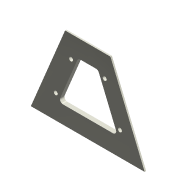
# Autodesk Inventor part: Stage2
Saved by Autodesk Inventor 2018.2 (Build 222227000, 227)
## iProperties
Created: 2018-11-01
Part Number: Stage2
Material: ABS-Kunststoff
Document SubType Name: Modeling
Designer: M.Knabel
Density: 1.06 g/cm^3
Appearance: Glatt - Elfenbein
Mass: 26.953 g
Surface Area: 131.178 cm^2
Volume: 25.4274 cm^3
Author: M.Knabel
Autodesk Inventor part; units mm, degrees
ref_plane "YZ Plane" through (0, 0, 0) normal (1, 0, 0) x (0, 1, 0)
ref_plane "XZ Plane" through (0, 0, 0) normal (0, 1, 0) x (-1, 0, 0)
ref_plane "XY Plane" through (0, 0, 0) normal (0, 0, 1) x (1, 0, 0)
sketch "Skizze1" plane through (0, 0, 0) normal (0, 1, 0) x (-1, 0, 0)
  line L0 (-22.75, 41.5) -> (22.75, 41.5)
  line L1 (22.75, 41.5) -> (57.1297, -41.5)
  line L2 (57.1297, -41.5) -> (-57.1297, -41.5)
  line L3 (-57.1297, -41.5) -> (-22.75, 41.5)
  line L4 (79.9816, 0) -> (-79.9816, 0) construction
  line L5 (0, -58.1) -> (0, 58.1) construction
  point P0 (0, 0)
  dimension "d0" = 83
  dimension "d1" = 112.5
  dimension "d2" = 45.5
  constraints: 8 end point, 1 horizontal, 1 parallel, 2 other
  measures "d0" distance between parallel lines of L2 L0
  measures "d1" angle of L0 L3
  measures "d2" distance of L0.start L0.end
extrude "Extrusion1" add sketch "Skizze1" along normal blind 6
sketch "Skizze2" plane through (0, 6, 0) normal (0, 1, 0) x (1, 0, 0)
  line L0 (-22.75, -41.5) -> (22.75, -41.5) projected
  line L1 (22.75, -41.5) -> (57.1297, 41.5) projected
  line L2 (57.1297, 41.5) -> (-57.1297, 41.5) projected
  line L3 (-57.1297, 41.5) -> (-22.75, -41.5) projected
  line L4 (-49.6467, 36.5) -> (49.6467, 36.5)
  line L5 (49.6467, 36.5) -> (19.4091, -36.5)
  line L6 (19.4091, -36.5) -> (-19.4091, -36.5)
  line L7 (-19.4091, -36.5) -> (-49.6467, 36.5)
  point P0 (0, 0)
  dimension "d5" = 5
  constraints: 8 end point, 3 other
  measures "d5" distance between parallel lines of L2 L4
extrude "Extrusion2" cut sketch "Skizze2" against normal blind 3.5
sketch "Skizze4" plane through (0, 6, 0) normal (0, 1, 0) x (1, 0, 0)
  line L0 (58.5766, 41.5) -> (-55.8797, 41.5) construction
  line L1 (-55.8797, 41.5) -> (-21.5, -41.5) construction
  line L2 (-21.5, -41.5) -> (24.1969, -41.5) construction
  line L3 (57.1297, 41.5) -> (22.75, -41.5) construction
  line L4 (22.4292, -40.7678) -> (56.8089, 42.2322) construction
  line L5 (-29.4207, 23.8207) -> (30.0466, 23.8207)
  line L6 (30.0466, 23.8207) -> (10.313, -23.8207)
  line L7 (10.313, -23.8207) -> (-9.687, -23.8207)
  line L8 (-9.687, -23.8207) -> (-29.4207, 23.8207)
  point P0 (0, 0)
  dimension "d15" = 20
  constraints: 8 end point, 3 other
  measures "d15" distance of L6.end L7.end
extrude "Extrusion3" cut sketch "Skizze4" against normal through all
fillet "Rundung1" radius 3 4 edges at (30.0466, 3, -23.8207) (10.313, 3, 23.8207) (-9.687, 3, 23.8207) (-29.4207, 3, -23.8207)
sketch "Skizze5" plane through (0, 6, 0) normal (0, 1, 0) x (1, 0, 0)
  line L0 (-10.4541, -21.9687) -> (-27.7025, 19.6726) projected
  arc A0 (-24.9309, 23.8207) -> (-27.7025, 19.6726) centre (-24.9309, 20.8207) ccw projected
  line L1 (-24.9309, 23.8207) -> (25.5568, 23.8207) projected
  arc A1 (28.3284, 19.6726) -> (25.5568, 23.8207) centre (25.5568, 20.8207) ccw projected
  line L2 (28.3284, 19.6726) -> (11.0801, -21.9687) projected
  arc A2 (8.3084, -23.8207) -> (11.0801, -21.9687) centre (8.3084, -20.8207) ccw projected
  line L3 (8.3084, -23.8207) -> (-7.6825, -23.8207) projected
  arc A3 (-10.4541, -21.9687) -> (-7.6825, -23.8207) centre (-7.6825, -20.8207) ccw projected
  line L4 (-49.6467, 36.5) -> (-19.4091, -36.5) projected
  line L5 (-19.4091, -36.5) -> (19.4091, -36.5) projected
  line L6 (19.4091, -36.5) -> (49.6467, 36.5) projected
  line L7 (49.6467, 36.5) -> (-49.6467, 36.5) projected
  point P0 (0, 0)
extrude "Extrusion4" cut sketch "Skizze5" against normal blind 0.5
sketch "Skizze6" plane through (0, 5.5, 0) normal (0, 1, 0) x (1, 0, 0)
  circle A0 centre (-32.1216, 17.5) radius 4.7 construction
  circle A1 centre (-16.7957, -19.5) radius 4.7 construction
  circle A2 centre (16.9926, -19.5) radius 4.7 construction
  circle A3 centre (32.3185, 17.5) radius 4.7 construction
  line L0 (-24.9683, -43.2) -> (25.1652, -43.2) construction
  line L1 (25.1652, -43.2) -> (61.3675, 44.2) construction
  line L2 (61.3675, 44.2) -> (11.1438, 44.2) construction
  arc A4 (11.1438, 44.2) -> (-10.9469, 44.2) centre (0.0985, 34.5) ccw construction
  line L3 (-10.9469, 44.2) -> (-61.1705, 44.2) construction
  line L4 (-61.1705, 44.2) -> (-24.9683, -43.2) construction
  point P0 (0, 0)
  point P1 (-32.1216, 17.5)
  point P2 (-16.7957, -19.5)
  point P3 (16.9926, -19.5)
  point P4 (32.3185, 17.5)
  constraints: 4 coincident
hole "Bohrung2" at (-32.1216, 5.5, -17.5) at (-16.7957, 5.5, 19.5) at (16.9926, 5.5, 19.5) at (32.3185, 5.5, -17.5) direction (0, -1, 0) diameter 4 depth 8 tip angle 118
sketch "Skizze7" plane through (0, 5.5, 0) normal (0, 1, 0) x (1, 0, 0)
  circle A0 centre (16.9926, -19.5) radius 2 projected
  circle A1 centre (-32.1216, 17.5) radius 2 projected
  circle A2 centre (-16.7957, -19.5) radius 2 projected
  circle A3 centre (32.3185, 17.5) radius 2 projected
  arc A4 (-10.4541, -21.9687) -> (-7.6825, -23.8207) centre (-7.6825, -20.8207) ccw projected
  line L0 (-27.7025, 19.6726) -> (-10.4541, -21.9687) projected
  arc A5 (-24.9309, 23.8207) -> (-27.7025, 19.6726) centre (-24.9309, 20.8207) ccw projected
  line L1 (25.5568, 23.8207) -> (-24.9309, 23.8207) projected
  arc A6 (28.3284, 19.6726) -> (25.5568, 23.8207) centre (25.5568, 20.8207) ccw projected
  line L2 (11.0801, -21.9687) -> (28.3284, 19.6726) projected
  arc A7 (8.3084, -23.8207) -> (11.0801, -21.9687) centre (8.3084, -20.8207) ccw projected
  line L3 (-7.6825, -23.8207) -> (8.3084, -23.8207) projected
  line L4 (-19.4091, -36.5) -> (-49.6467, 36.5) projected
  line L5 (19.4091, -36.5) -> (-19.4091, -36.5) projected
  line L6 (49.6467, 36.5) -> (19.4091, -36.5) projected
  line L7 (-49.6467, 36.5) -> (49.6467, 36.5) projected
  point P0 (0, 0)
extrude "Extrusion5" cut sketch "Skizze7" against normal blind 1
fillet "Rundung2" radius 20 4 edges at (-19.4091, 3.5, 36.5) (19.4091, 3.5, 36.5) (49.6467, 3.5, -36.5) (-49.6467, 3.5, -36.5)
sketch "Skizze8" plane through (0, 2.5, 0) normal (0, 1, 0) x (1, 0, 0)
  line L0 (19.7146, 36.5) -> (-19.7146, 36.5) projected
  arc A0 (38.1922, 8.8463) -> (19.7146, 36.5) centre (19.7146, 16.5) ccw projected
  line L1 (24.5231, -24.1537) -> (38.1922, 8.8463) projected
  arc A1 (6.0455, -36.5) -> (24.5231, -24.1537) centre (6.0455, -16.5) ccw projected
  line L2 (-6.0455, -36.5) -> (6.0455, -36.5) projected
  arc A2 (-24.5231, -24.1537) -> (-6.0455, -36.5) centre (-6.0455, -16.5) ccw projected
  line L3 (-38.1922, 8.8463) -> (-24.5231, -24.1537) projected
  arc A3 (-19.7146, 36.5) -> (-38.1922, 8.8463) centre (-19.7146, 16.5) ccw projected
  line L4 (22.75, -41.5) -> (-22.75, -41.5) projected
  line L5 (57.1297, 41.5) -> (22.75, -41.5) projected
  line L6 (-57.1297, 41.5) -> (57.1297, 41.5) projected
  line L7 (-22.75, -41.5) -> (-57.1297, 41.5) projected
  point P0 (0, 0)
extrude "Extrusion6" cut sketch "Skizze8" against normal blind 1
